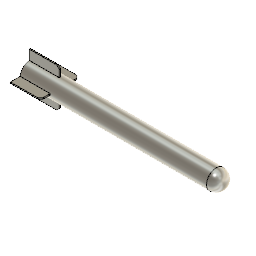
new solid thrusters v1 (Autodesk Fusion 360 design; units mm, degrees)
Autodesk Fusion 360 part; units mm, degrees
sketch "Sketch1" plane through (0, 0, 0) normal (0, 1, 0) x (1, 0, 0)
  line L0 (0, 0) -> (285, 0)
  arc A0 (285, 0) -> (300, 15) centre (285, 15) ccw
  line L1 (0, 2) -> (285, 2)
  arc A1 (285, 2) -> (298, 15) centre (285, 15) ccw
  line L2 (0, 2) -> (0, 0)
  line L3 (300, 15) -> (298, 15)
  dimension "d1" = 285
  constraint coincident L0.start L2.end
  constraint horizontal L0
  constraint tangent L0 A0
  constraint perpendicular L0 L2
  constraint concentric A0 A1
  constraint tangent L1 A1
  measures "d1" distance of L0.start L0.end
revolve "Revolve1" add sketch "Sketch1" angle 360 about axis through (300, 0, -15) along (-1, 0, 0) makes body 1
sketch "Sketch2" plane through (0, 0, 0) normal (0, 1, 0) x (1, 0, 0)
  line L0 (0, 0) -> (46, 0)
  line L1 (46, 0) -> (46, -11)
  line L2 (42, -15) -> (0, -15)
  line L3 (0, -15) -> (0, 0)
  line L4 (42, -15) -> (46, -11)
  dimension "d6" = 46
  dimension "d7" = 15
  dimension "d8" = 45
  dimension "d9" = 4
  constraint horizontal L0
  constraint vertical L1
  constraint horizontal L2
  constraint vertical L3
  constraint coincident L0.start L3.end
  measures "d6" distance of L0.start L0.end
  measures "d7" distance of L0.start L2.end
  measures "d8" angle of L2 L4
  measures "d9" horizontal distance of L2.start L1.end
extrude "Extrude1" add sketch "Sketch2" along normal mid plane 2 separate body makes body 2
pattern_circular "C-Pattern1" count 4 over 360 about axis through (300, 0, -15) along (-1, 0, 0) of bodies 2 makes body 3 at (29.3333, 20, -16) makes body 4 at (29.3333, -1, -35) makes body 5 at (29.3333, -20, -14)
